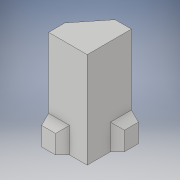
# Autodesk Inventor part: WheelIntakeBrace
Saved by Autodesk Inventor 2017 (Build 210142000, 142)
## iProperties
Created: 2017-12-16
Part Number: WheelIntakeBrace
Material: Generic
Document SubType Name: Modeling
Designer: User
Density: 1 g/cm^3
Appearance: Default
Author: User
Autodesk Inventor part; units mm, degrees
ref_plane "YZ Plane" through (0, 0, 0) normal (1, 0, 0) x (0, 1, 0)
ref_plane "XZ Plane" through (0, 0, 0) normal (0, 1, 0) x (-1, 0, 0)
ref_plane "XY Plane" through (0, 0, 0) normal (0, 0, 1) x (1, 0, 0)
sketch "Sketch1" plane through (0, 0, 0) normal (1, 0, 0) x (0, 1, 0)
  line L0 (0, 0) -> (65.278, 0)
  line L1 (65.278, 0) -> (65.278, -16.1544)
  line L2 (0, -16.1544) -> (0, 0)
  line L3 (0, 0) -> (0, -20.066)
  line L4 (65.278, 0) -> (0, 0)
  line L5 (0, 0) -> (0, -30.1625)
  line L6 (0, -30.1625) -> (65.278, -30.1625)
  line L7 (65.278, -30.1625) -> (65.278, 0)
  dimension "d0" = 65.278
  dimension "d1" = 16.1544
  dimension "d11" = 30.1625
  constraints: 16 end point, 3 parallel, 2 horizontal, 2 perpendicular, 1 point on line
  measures "d0" distance of L1.end L2.start
  measures "d1" distance of L0.end L1.end
  measures "d11" distance of L5.end L4.end
extrude "Extrusion1" add sketch "Sketch1" along normal blind 4.7625
sketch "Sketch3" plane through (0, 0, 0) normal (0, 0, 1) x (1, 0, 0)
  line L0 (0, 65.278) -> (0, 0) projected
  line L1 (0, 0) -> (4.7625, 0) projected
  line L2 (4.7625, 65.278) -> (4.7625, 0) projected
  line L3 (0, 65.278) -> (4.7625, 65.278) projected
  line L4 (4.7625, 65.278) -> (4.7625, 0) projected
  line L5 (4.7625, 65.278) -> (-21.59, 65.278)
  line L6 (-21.59, 65.278) -> (-21.59, 0)
  line L7 (-21.59, 0) -> (4.7625, 0)
  line L8 (4.7625, 0) -> (4.7625, 65.278)
  dimension "d12" = 26.3525
  constraints: 8 end point, 2 parallel, 1 horizontal, 1 perpendicular
  measures "d12" distance of L7.end L6.end
extrude "Extrusion3" add sketch "Sketch3" against normal blind 4.7625 contours L0 L7 L6 L5
sketch "Sketch4" plane through (0, 65.278, -30.1625) normal (0, 1, 0) x (1, 0, 0)
  line L0 (0, 0) -> (0, -25.4) projected
  line L1 (-21.59, -25.4) -> (0, -25.4) projected
  line L2 (-21.59, -30.1625) -> (-21.59, -25.4) projected
  line L3 (4.7625, -30.1625) -> (-21.59, -30.1625) projected
  line L4 (4.7625, 0) -> (4.7625, -30.1625) projected
  line L5 (0, 0) -> (4.7625, 0) projected
  line L6 (-21.59, -25.4) -> (0, -25.4) projected
  line L7 (-21.59, -25.4) -> (-21.59, -19.05)
  line L8 (0, 0) -> (-6.35, 0)
  line L9 (-6.35, 0) -> (-21.59, -19.05)
  point P0 (0, -30.1625)
  dimension "d15" = 6.35
  dimension "d16" = 6.35
  constraints: 6 end point, 1 horizontal, 1 vertical
  measures "d15" distance of L1.start L7.end
  measures "d16" distance of L0.start L8.end
extrude "Extrusion4" add sketch "Sketch4" against normal blind 4.7625 contours L0 L1 L7 L9 L8
fillet "Fillet1" radius 1.5875 3 edges at (0, 60.5155, -17.4625) (-10.795, 60.5155, -4.7625) (0, 30.2578, -4.7625)
sketch "Sketch6" plane through (0, 0, -30.1625) normal (0, -1, 0) x (1, 0, 0)
  line L0 (0, 23.8125) -> (0, 0) projected
  line L1 (0, 0) -> (4.7625, 0) projected
  line L2 (4.7625, 30.1625) -> (4.7625, 0) projected
  line L3 (-21.59, 30.1625) -> (4.7625, 30.1625) projected
  line L4 (-21.59, 30.1625) -> (-21.59, 25.4) projected
  line L5 (-1.5875, 25.4) -> (-21.59, 25.4) projected
  arc A0 (0, 23.8125) -> (-1.5875, 25.4) centre (-1.5875, 23.8125) ccw projected
  line L6 (0, 0) -> (9.525, 0)
  line L7 (9.525, 0) -> (9.525, 9.525)
  line L8 (9.525, 9.525) -> (0, 9.525)
  line L9 (0, 9.525) -> (0, 0)
  line L10 (-21.59, 30.1625) -> (-21.59, 25.4) projected
  line L11 (-21.59, 25.4) -> (-12.065, 25.4)
  line L12 (-12.065, 25.4) -> (-12.065, 34.925)
  line L13 (-12.065, 34.925) -> (-21.59, 34.925)
  line L14 (-21.59, 34.925) -> (-21.59, 25.4)
  point P0 (0, 30.1625)
  dimension "d24" = 9.525
  dimension "d25" = 9.525
  dimension "d26" = 9.525
  dimension "d27" = 9.525
  constraints: 16 end point, 4 parallel, 2 horizontal, 2 perpendicular
  measures "d24" distance of L8.end L7.end
  measures "d25" distance of L7.end L6.end
  measures "d26" distance of L13.end L12.end
  measures "d27" distance of L12.end L11.end
extrude "Extrusion5" add sketch "Sketch6" against normal blind 12.7 contours L8 L2 L1 L0 | L8 L7 L6 L2 | L5 L4 L3 L12 | L3 L14 L13 L12
chamfer "Chamfer1" distance 4.7625 angle 45 4 edges at (4.7625, 6.35, -20.6375) (-12.065, 6.35, 0) (4.7625, 12.7, -25.4) (-16.8275, 12.7, 0)
body "Solid1"
